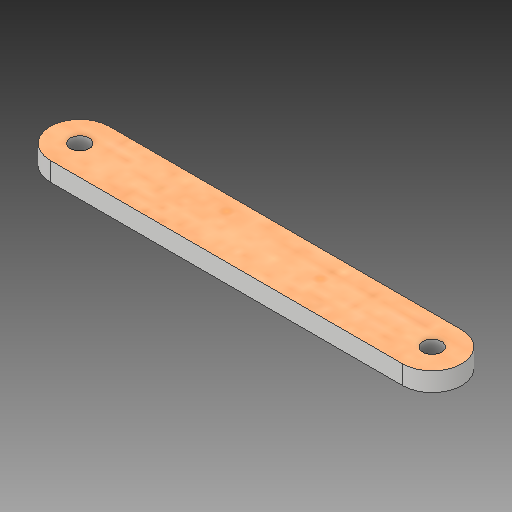
# Autodesk Inventor part: portabateria
Saved by Autodesk Inventor 2018 (Build 220112000, 112)
## iProperties
Created: 2017-05-11
Part Number: portabateria
Material: Generic
Document SubType Name: Modeling
Designer: Vidal Villegas
Density: 1 g/cm^3
Appearance: Default
Mass: 2.11204 g
Surface Area: 18.6733 cm^2
Volume: 2.11204 cm^3
Author: Vidal Villegas
Autodesk Inventor part; units mm, degrees
ref_plane "YZ Plane" through (0, 0, 0) normal (1, 0, 0) x (0, 1, 0)
ref_plane "XZ Plane" through (0, 0, 0) normal (0, 1, 0) x (-1, 0, 0)
ref_plane "XY Plane" through (0, 0, 0) normal (0, 0, 1) x (1, 0, 0)
sketch "Sketch1" plane through (0, 0, 0) normal (0, 1, 0) x (-1, 0, 0)
  circle A0 centre (59.7558, 0) radius 1.6
  circle A1 centre (0, 0) radius 1.6
  arc A2 (59.7558, -5) -> (59.7558, 5) centre (59.7558, 0) ccw
  arc A3 (0, 5) -> (0, -5) centre (0, 0) ccw
  line L0 (59.7558, 5) -> (0, 5)
  line L1 (59.7558, -5) -> (0, -5)
  dimension "d0" = 3.2
  dimension "d1" = 3.2
  dimension "d2" = 59.7557
  dimension "d12" = 10
  dimension "d13" = 10
  constraints: 4 centre point, 4 coincident, 4 end point, 4 point on circle, 2 horizontal, 2 tangent, 1 equal radius, 1 horizontal alignment
  measures "d0" diameter of A0
  measures "d1" diameter of A1
  measures "d2" distance of A1.centre A0.centre
  measures "d12" diameter of A2
  measures "d13" diameter of A3
extrude "Extrusion1" add sketch "Sketch1" along normal blind 3.2
equation "\"d13\" = d12"
body "Solid1"
